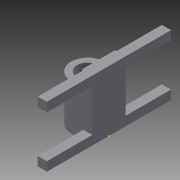
# Autodesk Inventor part: Slider
Saved by Autodesk Inventor 2015 (Build 190159000, 159)
## iProperties
Created: 2016-05-27
Part Number: Slider
Material: Generic
Document SubType Name: Modeling
Designer: Toby
Density: 1 g/cm^3
Appearance: Default
Author: Toby
Autodesk Inventor part; units mm, degrees
ref_plane "YZ Plane" through (0, 0, 0) normal (1, 0, 0) x (0, 1, 0)
ref_plane "XZ Plane" through (0, 0, 0) normal (0, 1, 0) x (-1, 0, 0)
ref_plane "XY Plane" through (0, 0, 0) normal (0, 0, 1) x (1, 0, 0)
sketch "Sketch1" plane through (0, 0, 0) normal (0, 0, 1) x (1, 0, 0)
  circle A0 centre (0, 0) radius 5.5
  line L0 (0, 5.5) -> (11.9603, 5.5)
  line L1 (11.9603, 5.5) -> (11.9603, -5.5)
  line L2 (11.9603, -5.5) -> (0, -5.5)
  line L3 (0, -5.5) -> (0, 5.5)
  circle A1 centre (0, 0) radius 3.5
  dimension "d1" = 11
  dimension "d0" = 7
  dimension "d2" = 11
  constraints: 8 end point, 2 coincident, 2 parallel, 1 centre point, 1 horizontal, 1 perpendicular, 1 vertical alignment, 2 other
  measures "d0" diameter of A1
  measures "d2" distance between parallel lines of L2 L0
extrude "Extrusion1" add sketch "Sketch1" along normal blind 15 contours A0 L3 A1 | A0 L0 L1 L2 | L3 A1 A0 | A1 L3 picked at (0.9121, 0.7274)
sketch "Sketch2" plane through (0, 0, 15) normal (0, 0, 1) x (1, 0, 0)
  circle A0 centre (0, 0) radius 3.5
  constraints: 1 centre point, 1 coincident
extrude "Extrusion2" cut sketch "Sketch2" against normal blind 15
sketch "Sketch3" plane through (0, 0, 15) normal (0, 0, 1) x (1, 0, 0)
  line L0 (11.9603, -5.5) -> (0, -5.5) projected
  line L1 (7, 5.5) -> (11.9603, 5.5)
  line L2 (11.9603, 5.5) -> (11.9603, -5.5)
  line L3 (11.9603, -5.5) -> (7, -5.5)
  line L4 (7, -5.5) -> (7, 5.5)
  line L5 (11.9603, -5.5) -> (11.9603, 5.5) projected
  line L6 (11.9603, 5.5) -> (0, 5.5) projected
  point P0 (0, 0)
  dimension "d7" = 7
  dimension "d8" = 0
  dimension "d9" = 0
  constraints: 8 end point, 2 parallel, 1 horizontal, 1 perpendicular, 1 point on line
  measures "d7" distance from line of point (0, 0) L4
  measures "d8" distance between parallel lines of L5 L2
  measures "d9" distance between parallel lines of L6 L1
extrude "Extrusion3" cut sketch "Sketch3" against normal blind 15
sketch "Sketch4" plane through (7, -5.5, 15) normal (1, 0, 0) x (0, 0, -1)
  point P0 (15, 5.5)
sketch "Sketch5" plane through (0, 0, 15) normal (0, 0, 1) x (1, 0, 0)
  point P0 (0, 0)
sketch "Sketch6" plane through (0, 0, 15) normal (0, 0, 1) x (1, 0, 0)
  line L0 (7, -5.5) -> (0, -5.5) projected
  line L1 (7, 5.5) -> (3.5, 5.5)
  line L2 (3.5, 5.5) -> (3.5, -5.5)
  line L3 (3.5, -5.5) -> (7, -5.5)
  line L4 (7, -5.5) -> (7, 5.5)
  point P0 (0, 0)
  constraints: 8 end point, 2 parallel, 1 horizontal, 1 midpoint, 1 perpendicular
extrude "Extrusion4" add sketch "Sketch6" along normal blind 5
sketch "Sketch7" plane through (7, -5.5, 0) normal (1, 0, 0) x (0, 0, -1)
  line L0 (-3, -15) -> (0, -15)
  line L1 (0, -15) -> (0, 26)
  line L2 (0, 26) -> (-3, 26)
  line L3 (-3, 26) -> (-3, -15)
  line L4 (-20, -15) -> (-17, -15)
  line L5 (-17, -15) -> (-17, 26)
  line L6 (-17, 26) -> (-20, 26)
  line L7 (-20, 26) -> (-20, -15)
  line L8 (-20, 0) -> (-20, 11) projected
  line L9 (0, 0) -> (-20, 0) projected
  line L10 (-20, 11) -> (0, 11) projected
  point P0 (0, 5.5)
  dimension "d14" = 3
  dimension "d15" = 20
  dimension "d16" = 3
  dimension "d17" = 0
  dimension "d18" = 15
  dimension "d19" = 15
  dimension "d20" = 41
  constraints: 16 end point, 4 parallel, 2 horizontal, 2 perpendicular, 2 point on line
  measures "d14" distance between parallel lines of L5 L7
  measures "d15" distance between parallel lines of L1 L7
  measures "d16" distance of L0.start L0.end
  measures "d17" distance between parallel lines of L8 L7
  measures "d18" distance between parallel lines of L9 L4
  measures "d19" distance between parallel lines of L10 L6
  measures "d20" distance of L6.end L4.start
extrude "Extrusion5" add sketch "Sketch7" against normal blind 3 contours L3 L9 L1 L0 | L3 L10 L1 L9 | L3 L2 L1 L10 | L9 L7 L10 L5 | L5 L4 L7 L9 | L10 L7 L6 L5
body "Solid1"
